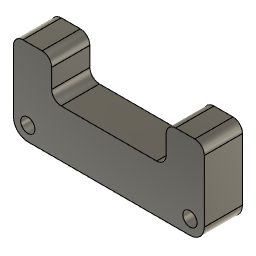
Part 1 (Autodesk Fusion 360 design; units mm, degrees)
part number: Tutorial Part 1
Autodesk Fusion 360 part; units mm, degrees
sketch "Sketch1" plane through (0, 0, 0) normal (0, 1, 0) x (1, 0, 0)
  line L0 (-137.3579, 25) -> (62.6421, 25)
  line L1 (62.6421, 25) -> (62.6421, -65)
  line L2 (-137.3579, -65) -> (-137.3579, 25)
  line L3 (-97.3579, -65) -> (-97.3579, -25)
  line L4 (-97.3579, -25) -> (22.6421, -25)
  line L5 (22.6421, -25) -> (22.6421, -65)
  line L6 (62.6421, -65) -> (22.6421, -65)
  line L7 (-97.3579, -65) -> (-137.3579, -65)
  dimension "d1" = 200
  dimension "d2" = 90
  dimension "d8" = 50
  constraint horizontal L0
  constraint vertical L1
  constraint horizontal L6
  constraint vertical L2
  constraint coincident L3.start L6
  constraint perpendicular L3 L6
  constraint perpendicular L3 L4
  constraint perpendicular L5 L6
  constraint collinear L6 L7
  measures "d1" distance of L1.end L2.start
  measures "d2" distance of L0.end L1.end
  measures "d8" distance of L0 L4
extrude "Extrude1" add sketch "Sketch1" along normal blind 40
fillet "Fillet1" radius 10 6 edges at (-137.3579, 20, 65) (-97.3579, 20, 65) (-97.3579, 20, 25) (22.6421, 20, 25) (22.6421, 20, 65) (62.6421, 20, 65)
fillet "Fillet2" radius 15 2 edges at (-137.3579, 20, -25) (62.6421, 20, -25)
sketch "Sketch2" plane through (0, 0, 0) normal (0, -1, 0) x (1, 0, 0)
  arc A0 (47.6421, -25) -> (62.6421, -10) centre (47.6421, -10) ccw
  line L0 (62.6421, -10) -> (62.6421, 55)
  arc A1 (62.6421, 55) -> (52.6421, 65) centre (52.6421, 55) ccw
  line L1 (52.6421, 65) -> (32.6421, 65)
  arc A2 (32.6421, 65) -> (22.6421, 55) centre (32.6421, 55) ccw
  line L2 (22.6421, 55) -> (22.6421, 35)
  arc A3 (12.6421, 25) -> (22.6421, 35) centre (12.6421, 35) ccw
  line L3 (12.6421, 25) -> (-87.3579, 25)
  arc A4 (-97.3579, 35) -> (-87.3579, 25) centre (-87.3579, 35) ccw
  line L4 (-97.3579, 35) -> (-97.3579, 55)
  arc A5 (-97.3579, 55) -> (-107.3579, 65) centre (-107.3579, 55) ccw
  line L5 (-107.3579, 65) -> (-127.3579, 65)
  arc A6 (-127.3579, 65) -> (-137.3579, 55) centre (-127.3579, 55) ccw
  line L6 (-137.3579, 55) -> (-137.3579, -10)
  arc A7 (-137.3579, -10) -> (-122.3579, -25) centre (-122.3579, -10) ccw
  line L7 (-122.3579, -25) -> (47.6421, -25)
  circle A8 centre (-122.3579, -10) radius 7.5
  circle A9 centre (47.6421, -10) radius 7.5
  dimension "d13" = 15
  dimension "d14" = 15
  constraint concentric A7 A8
  constraint concentric A0 A9
  measures "d13" diameter of A8
  measures "d14" diameter of A9
extrude "Extrude2" cut sketch "Sketch2" against normal blind 40 contours A8 | A9
